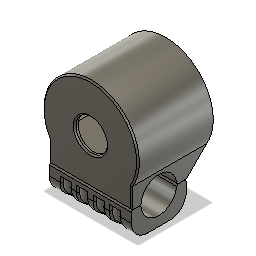
Emergency Button Case v2 (Autodesk Fusion 360 design; units mm, degrees)
Autodesk Fusion 360 part; units mm, degrees
box "BoxPrimitive1" add length 35 width 60 height 55 placed x (0, 1, 0) y (-1, 0, 0) z (0, 0, 1) at (60, 0, 0) makes body 1
sketch "Sketch2" plane through (0, 0, 55) normal (0, 0, 1) x (1, 0, 0)
  line L0 (60, 35) -> (0, 35)
  line L1 (0, 35) -> (0, 0)
  line L2 (0, 0) -> (60, 0)
  line L3 (60, 0) -> (60, 35)
  circle A0 centre (30, 17.5) radius 34.7311
  constraint coincident L1.end A0
  constraint coincident L0.start A0
  constraint coincident L2.end A0
extrude "Extrude1" add sketch "Sketch2" against normal blind 55 contours L3 A0 | L0 A0 | L1 A0 bodies 1
shell "Shell1" thickness 3 removed faces 1 at (26.5805, 16.8939, 0) on bodies 1
sketch "Sketch3" plane through (0, 0, 55) normal (0, 0, 1) x (1, 0, 0)
  line L0 (0, 0) -> (60, 0)
  arc A0 (60, 0) -> (0, 0) centre (30, 17.5) ccw
  line L1 (0, 0) -> (60, 0)
  line L2 (60, 0) -> (60, 35)
  line L3 (60, 35) -> (0, 35)
  line L4 (0, 35) -> (0, 0)
  circle A1 centre (30, 17.5) radius 11.5
  dimension "d10" = 23
  constraint horizontal L1
  constraint vertical L2
  constraint horizontal L3
  constraint vertical L4
  constraint coincident A0 L2.end
  constraint coincident L0.start A0.end
  constraint coincident L0.end A0.start
  constraint concentric A0 A1
  measures "d10" diameter of A1
extrude "Extrude2" cut sketch "Sketch3" against normal blind 3 contours A1 bodies 1
sketch "Sketch4" plane through (0, 0, 0) normal (1, 0, 0) x (0, 0, -1)
  circle A0 centre (-35, -15) radius 13
  circle A1 centre (-35, -15) radius 20
  line L0 (-55, 0) -> (-55, -15)
  line L1 (0, 0) -> (-15, -15)
  line L2 (-55, -15) -> (-15, -15)
  line L3 (0, 0) -> (-55, 0)
  point P0 (-55, 0)
  dimension "d13" = 26
  dimension "d14" = 40
  dimension "d15" = 15
  constraint concentric A0 A1
  constraint vertical L0
  constraint coincident P0 L0.start
  constraint coincident A1 L0.end
  constraint tangent A1 L0
  constraint coincident L1.start L3.start
  constraint coincident A1 L1.end
  constraint perpendicular L0 L2
  measures "d13" diameter of A0
  measures "d14" diameter of A1
  measures "d15" vertical distance of L1.start A0.centre
extrude "Extrude3" add sketch "Sketch4" along normal blind 60 contours A0 A1 L2 L3 | A1 L1 L3 | A1 L0 L3 bodies 1
sketch "Sketch5" plane through (0, -15, 0) normal (0, -1, 0) x (1, 0, 0)
  line L0 (0, 55) -> (0, 48)
  line L1 (0, 48) -> (60, 48)
  line L2 (60, 48) -> (60, 55)
  line L3 (60, 55) -> (0, 55)
  line L4 (0, 51.5) -> (60, 51.5) construction
  circle A0 centre (12, 51.5) radius 1.1
  circle A1 centre (24, 51.5) radius 1.1
  circle A2 centre (36, 51.5) radius 1.1
  circle A3 centre (48, 51.5) radius 1.1
  line L5 (0, 48) -> (60, 48)
  line L6 (60, 48) -> (60, 35)
  line L7 (60, 35) -> (0, 35)
  line L8 (0, 35) -> (0, 48)
  circle A4 centre (12, 18.5) radius 1.1
  circle A5 centre (24, 18.5) radius 1.1
  circle A6 centre (36, 18.5) radius 1.1
  circle A7 centre (48, 18.5) radius 1.1
  dimension "d18" = 12
  dimension "d19" = 12
  dimension "d20" = 12
  dimension "d21" = 12
  dimension "d22" = 2.2
  dimension "d23" = 60
  dimension "d24" = 13
  constraint midpoint L0 L4.start
  constraint midpoint L2 L4.end
  constraint coincident L4 A0.centre
  constraint coincident L4 A1.centre
  constraint coincident L4 A2.centre
  constraint coincident L4 A3.centre
  constraint equal A1 A2
  constraint equal A2 A3
  constraint equal A0 A1
  constraint horizontal L5
  constraint vertical L6
  constraint horizontal L7
  constraint vertical L8
  constraint coincident L0.end L1.start
  constraint symmetric A0 L7 A4
  constraint symmetric A1 L7 A5
  constraint symmetric A2 L7 A6
  constraint symmetric A3 L7 A7
  measures "d18" distance of L4.start A0.centre
  measures "d19" distance of A0.centre A1.centre
  measures "d20" distance of A1.centre A2.centre
  measures "d21" distance of A2.centre A3.centre
  measures "d22" diameter of A0
  measures "d23" distance of L0.end L1.end
  measures "d24" distance of L0.end L7.end
extrude "Extrude4" cut sketch "Sketch5" against normal blind 15 contours A0 | A1 | A2 | A3 | A4 | A5 | A6 | A7 bodies 1
chamfer "Chamfer1" distance 1 angle 45 3 edges at (30, -15, 22) (30, -15, 48) (30, -15, 55) on bodies 1
chamfer "Chamfer2" distance 1 angle 45 4 edges at (0, -7, 55) (30, 52.2311, 55) (19.2782, 21.6586, 55) (60, -7, 55) on bodies 1
sketch "Sketch6" plane through (0, 0, 0) normal (-1, 0, 0) x (0, 0, 1)
  line L0 (54, -15) -> (54, 0)
  line L1 (54, 0) -> (0, 0)
  line L2 (0, 0) -> (15, -15)
  line L3 (15, -15) -> (21, -15)
  line L4 (21, -15) -> (22.0385, -14.0007)
  arc A0 (47.9615, -14.0007) -> (22.0385, -14.0007) centre (35, -15) ccw
  line L5 (47.9615, -14.0007) -> (49, -15)
  line L6 (49, -15) -> (54, -15)
  circle A1 centre (35, -15) radius 13
  circle A2 centre (35, -15) radius 20
  line L7 (15, -15) -> (55, -15)
  line L8 (55, -15) -> (55, -23)
  line L9 (43, -35) -> (27, -35)
  line L10 (15, -23) -> (15, -15)
  arc A3 (15, -23) -> (27, -35) centre (27, -23) ccw
  arc A4 (43, -35) -> (55, -23) centre (43, -23) ccw
  dimension "d29" = 40
  dimension "d30" = 12
  constraint concentric A0 A1
  constraint coincident A0.start A1
  constraint concentric A1 A2
  constraint horizontal L7
  constraint vertical L8
  constraint horizontal L9
  constraint vertical L10
  constraint coincident L2.end L3.start
  constraint tangent A2 L8
  constraint tangent A2 L9
  constraint tangent L9 A3
  constraint tangent L10 A3
  constraint tangent L8 A4
  constraint tangent L9 A4
  constraint equal A3 A4
  measures "d29" diameter of A2
  measures "d30" radius of A3
extrude "Extrude5" add sketch "Sketch6" against normal blind 60 separate body contours L3 L6 A1 A2 L7 | A2 L8 L9 A4 | A2 L9 L10 A3 makes body 2
chamfer "Chamfer3" distance 1 angle 45 4 edges at (30, -15, 22) (30, -15, 55) (30, -15, 48) (30, -15, 15) on bodies 2
chamfer "Chamfer4" distance 1 angle 45 1 edges at (30, -15, 15) on bodies 1
sketch "Sketch7" plane through (0, -15, 0) normal (0, -1, 0) x (1, 0, 0)
  circle A0 centre (24, 51.5) radius 1.1
  circle A1 centre (36, 51.5) radius 1.1
  circle A2 centre (12, 51.5) radius 1.1
  circle A3 centre (48, 51.5) radius 1.1
  line L0 (60, 54) -> (0, 54)
  line L1 (0, 54) -> (0, 49)
  line L2 (0, 49) -> (60, 49)
  line L3 (60, 49) -> (60, 54)
sketch "Sketch8" plane through (0, -15, 0) normal (0, -1, 0) x (1, 0, 0)
  circle A0 centre (36, 18.5) radius 1.1
  circle A1 centre (24, 18.5) radius 1.1
  circle A2 centre (48, 18.5) radius 1.1
  circle A3 centre (12, 18.5) radius 1.1
  line L0 (0, 16) -> (60, 16)
  line L1 (60, 16) -> (60, 21)
  line L2 (60, 21) -> (0, 21)
  line L3 (0, 21) -> (0, 16)
extrude "Extrude6" cut sketch "Sketch8" sketch "Sketch7" along normal blind 23 contours A0 | A1 | A2 | A3 of sketch 2 contours A0 | A1 | A2 | A3 bodies 2
sketch "Sketch9" plane through (0, -15, 0) normal (0, 1, 0) x (-1, 0, 0)
  circle A0 centre (-24, 51.5) radius 1.1
  circle A1 centre (-36, 51.5) radius 1.1
  circle A2 centre (-12, 51.5) radius 1.1
  circle A3 centre (-48, 51.5) radius 1.1
  line L0 (-60, 49) -> (0, 49)
  line L1 (0, 49) -> (0, 54)
  line L2 (0, 54) -> (-60, 54)
  line L3 (-60, 54) -> (-60, 49)
  circle A4 centre (-12, 51.5) radius 3.75
  circle A5 centre (-24, 51.5) radius 3.75
  circle A6 centre (-36, 51.5) radius 3.75
  circle A7 centre (-48, 51.5) radius 3.75
  circle A8 centre (-12, 18.5) radius 3.75
  circle A9 centre (-24, 18.5) radius 3.75
  circle A10 centre (-36, 18.5) radius 3.75
  circle A11 centre (-48, 18.5) radius 3.75
  dimension "d37" = 7.5
  dimension "d40" = -36
  dimension "d41" = -33
  constraint concentric A2 A4
  measures "d37" diameter of A4
extrude "Extrude7" cut sketch "Sketch9" against normal blind 36 from surface at -4 contours L0 L2 A7 | L0 A7 | L2 A7 | L0 L2 A6 | L0 A6 | L2 A6 | L0 L2 A5 | L0 A5 | L2 A5 | L0 L2 A4 | L0 A4 | L2 A4 | A8 | A9 | A10 | A11 bodies 2
fillet "Fillet1" radius 1 24 edges at (46.6537, -21, 15) (48, -34.0199, 22.25) (49.3463, -21, 15) (34.6537, -21, 15) (36, -34.0199, 22.25) (37.3463, -21, 15) (22.6537, -21, 15) (24, -34.0199, 22.25) (25.3463, -21, 15) (10.6537, -21, 15) (12, -34.0199, 22.25) (13.3463, -21, 15) (49.3463, -21, 55) (48, -34.0199, 47.75) (46.6537, -21, 55) (37.3463, -21, 55) (36, -34.0199, 47.75) (34.6537, -21, 55) (25.3463, -21, 55) (24, -34.0199, 47.75) (22.6537, -21, 55) (13.3463, -21, 55) (12, -34.0199, 47.75) (10.6537, -21, 55) on bodies 2
move_face "OffsetFaces1" offset -0.4 8 faces at (13.0945, -17.6667, 18.6095) (24.8768, -16.3333, 19.1642) (35.034, -16.3333, 19.0261) (48.5018, -16.3333, 19.4789) (49.0986, -17.6667, 51.4452) (37.0986, -17.6667, 51.4452) (25.0986, -17.6667, 51.4452) (13.0986, -17.6667, 51.4452) on bodies 2
move_face "OffsetFaces2" offset -0.5 1 faces at (28.1737, 42.364, 52) on bodies 1
sketch "Sketch10" plane through (0, 0, 52.5) normal (0, 0, -1) x (-1, 0, 0)
  circle A0 centre (-30, 17.5) radius 11.5
  line L0 (-58.2243, 3) -> (-1.7757, 3)
  arc A1 (-1.7757, 3) -> (-58.2243, 3) centre (-30, 17.5) ccw
  line L1 (-52.5, 39.8744) -> (-7.5, 39.8744)
  dimension "d49" = 45
  constraint coincident A1 L1.start
  constraint coincident A1 L1.end
  constraint horizontal L1
  measures "d49" distance of L1.start L1.end
extrude "Extrude8" add sketch "Sketch10" along normal blind 52.5 contours A1 L1 bodies 1
ref_plane "WorkPlane1" through (52.5, 39.8744, 26.25) normal (1, 0, 0) x (0, 0, -1)
ref_plane "WorkPlane2" through (30, 39.8744, 26.25) normal (1, 0, 0) x (0, 0, -1)
sketch "Sketch11" plane through (30, 39.8744, 26.25) normal (1, 0, 0) x (0, 0, -1)
  circle A0 centre (26.25, 0) radius 5
  circle A1 centre (26.25, 0) radius 8
  line L0 (26.25, -39.8744) -> (26.25, 12.3567)
  line L1 (-26.25, 0) -> (26.25, 0)
  dimension "d54" = 10
  dimension "d55" = 16
  constraint concentric A0 A1
  constraint coincident A0.centre L0
  constraint coincident A0.centre L1
  measures "d54" diameter of A0
  measures "d55" diameter of A1
extrude "Extrude9" cut sketch "Sketch11" along normal mid plane 6 contours A0 A1 L0 L1 picked at (19.2941, 0.6167) bodies 1
fillet "Fillet2" radius 1 2 edges at (30, 44.8744, 0) (30, 39.8744, 5) on bodies 1
